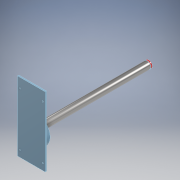
# Autodesk Inventor part: DecAxis
Saved by Autodesk Inventor 2022 (Build 260153000, 153)
## iProperties
Created: 2021-04-24
Part Number: DecAxis
Material: Generic
Document SubType Name: Modeling
Designer: Mick Veldhuis
Density: 1 g/cm^3
Appearance: Smooth - Black(1)
Mass: 1664.21 g
Surface Area: 2199.45 cm^2
Volume: 1664.21 cm^3
Author: Mick Veldhuis
Autodesk Inventor part; units mm, degrees
ref_plane "YZ Plane" through (0, 0, 0) normal (1, 0, 0) x (0, 1, 0)
ref_plane "XZ Plane" through (0, 0, 0) normal (0, 1, 0) x (-1, 0, 0)
ref_plane "XY Plane" through (0, 0, 0) normal (0, 0, 1) x (1, 0, 0)
sketch "Sketch1" plane through (0, 0, 0) normal (0, 0, 1) x (1, 0, 0)
  circle A0 centre (0, 0) radius 78
  constraints: 1 centre point, 1 coincident
extrude "Connector" add sketch "Sketch1" along normal blind 20
sketch "Sketch2" plane through (0, 0, 0) normal (0, 0, -1) x (-1, 0, 0)
  circle A0 centre (0, 0) radius 20
  constraints: 1 centre point, 1 coincident
extrude "RotAxis" add sketch "Sketch2" along normal blind 624
sketch "Sketch3" plane through (0, 0, 20) normal (0, 0, 1) x (1, 0, 0)
  line L0 (78, 234) -> (-78, 234)
  line L1 (-78, 234) -> (-78, -156)
  line L2 (-78, -156) -> (78, -156)
  line L3 (78, -156) -> (78, 234)
  point P0 (0, 0)
  constraints: 8 end point, 2 parallel, 1 horizontal, 1 perpendicular
extrude "TelescopeMount" add sketch "Sketch3" along normal blind 8
sketch "Sketch4" plane through (0, 0, -624) normal (0, 0, -1) x (-1, 0, 0)
  circle A0 centre (0, 0) radius 21
  constraints: 1 centre point, 1 coincident
extrude "Cap" add sketch "Sketch4" along normal blind 8
sketch "Sketch5" plane through (0, 0, 28) normal (0, 0, 1) x (1, 0, 0)
  line L0 (-78, 234) -> (-78, -156) projected
  line L1 (78, -156) -> (78, 234) projected
  point P0 (0, 0)
  point P1 (64, -120)
  point P2 (-64, -120)
  point P3 (-64, 180)
  point P4 (64, 180)
hole "Hole1" at (64, -120, 28) at (-64, -120, 28) at (-64, 180, 28) at (64, 180, 28) direction (0, 0, -1) diameter 6.647 end through all thread size "M8x1.25" class "6H" standard "ISO Metric profile"
body "Solid1"
